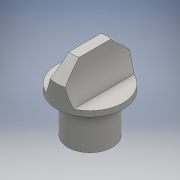
# Autodesk Inventor part: Arm - 608 bearing cap
Saved by Autodesk Inventor 2016 (Build 200138000, 138)
## iProperties
Created: 2016-05-11
Part Number: Arm - 608 bearing cap
Material: Generic
Document SubType Name: Modeling
Designer: alist
Density: 1 g/cm^3
Appearance: Default
Author: alist
Autodesk Inventor part; units mm, degrees
ref_plane "YZ Plane" through (0, 0, 0) normal (1, 0, 0) x (0, 1, 0)
ref_plane "XY Plane" through (0, 0, 0) normal (0, 0, 1) x (1, 0, 0)
sketch "Sketch1" plane through (0, 0, 0) normal (0, 0, 1) x (1, 0, 0)
  circle A0 centre (1.0409, 9.1519) radius 2.25 projected
  circle A1 centre (1.0409, 9.1519) radius 4
  point P0 (0, 0)
  dimension "d0" = 8
  constraints: 1 centre point, 1 coincident
  measures "d0" diameter of A1
extrude "Extrusion1" add sketch "Sketch1" along normal blind 1 contours A0 | A1
sketch "Sketch2" plane through (1.0409, 9.1519, 1) normal (0, 0, 1) x (1, 0, 0)
  circle A0 centre (0, 0) radius 4
  point P0 (-1.0409, -9.1519)
  dimension "d3" = 8
  constraints: 1 centre point
  measures "d3" diameter of A0
extrude "Extrusion2" add sketch "Sketch2" along normal blind 6
sketch "Sketch3" plane through (1.0409, 9.1519, 7) normal (0, 0, 1) x (1, 0, 0)
  circle A0 centre (0, 0) radius 6
  point P0 (-1.0409, -9.1519)
  dimension "d6" = 12
  constraints: 1 centre point
  measures "d6" diameter of A0
extrude "Extrusion3" add sketch "Sketch3" along normal blind 1
hole "Hole1" at (1.0409, 9.1519, 8) direction (0, 0, -1) diameter 3.9 end through all
sketch "Sketch4" plane through (1.0409, 9.1519, 8) normal (0, 0, 1) x (1, 0, 0)
  line L0 (2.5, 5.4544) -> (2.5, -5.4544)
  line L1 (-2.5, -5.4544) -> (-2.5, 5.4544)
  circle A0 centre (0, 0) radius 1.95 projected
  circle A1 centre (0, 0) radius 6 projected
  point P0 (-1.0409, -9.1519)
  dimension "d22" = 2.5
  dimension "d23" = 2.5
  constraints: 4 end point, 4 point on circle, 1 parallel
  measures "d22" distance from line of L1 A0.centre
  measures "d23" distance from line of L0 A0.centre
extrude "Extrusion4" add sketch "Sketch4" along normal blind 6 contours L0 A1 L1 | A0
ref_plane "Work Plane1" through (1.0409, 3.1519, 7) normal (0, 1, 0) x (-1, 0, 0)
sketch "Sketch5" plane through (1.0409, 3.1519, 7) normal (0, 1, 0) x (-1, 0, 0)
  line L0 (-2.5, 1) -> (-2.5, 1) projected
  line L1 (-2.5, 1) -> (-2.5, 7) projected
  line L2 (2.5, 7) -> (-2.5, 7) projected
  line L3 (2.5, 1) -> (2.5, 7) projected
  line L4 (2.5, 1) -> (2.5, 1) projected
  line L5 (2.5, 1) -> (2.5, 7) projected
  line L6 (-2.5, 7) -> (2.5, 7) projected
  line L7 (-2.5, 1) -> (-2.5, 7) projected
  line L8 (-6, 0) -> (6, 0) projected
  line L9 (6, 1) -> (2.5, 1) projected
  arc A0 (0.9, 7) -> (2.5, 1) centre (15.8796, 7.7812) ccw
  line L10 (2.5, 7) -> (-2.5, 7) projected
  line L11 (0, 7) -> (0, 0)
  line L12 (4, 0) -> (-4, 0) projected
  line L13 (-2.5, 1) -> (-6, 1) projected
  arc A1 (-2.5, 1) -> (-0.9, 7) centre (-15.8796, 7.7812) ccw
  point P0 (1.0409, -7)
  dimension "d26" = 15
  dimension "d27" = 15
  dimension "d28" = 1.8
  dimension "d29" = 1.8
  constraints: 4 point on circle, 2 centre point, 2 end point, 2 midpoint, 2 point on line
  measures "d26" radius of A0
  measures "d27" radius of A1
  measures "d28" diameter of A0.start L11
  measures "d29" diameter of A1.end L11
extrude "Extrusion5" cut sketch "Sketch5" along normal through all
chamfer "Chamfer1" distance 3 angle 45 2 edges at (1.0409, 3.1519, 14) (1.0409, 15.1519, 14)
equation "\"d23\" = d22"
equation "\"d29\" = d28"
body "Solid1"
